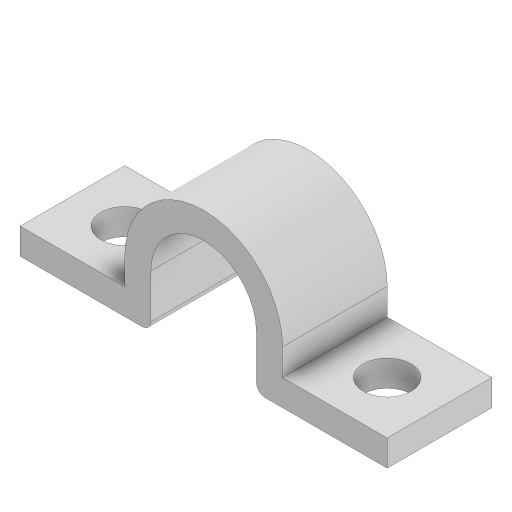
# Autodesk Inventor part: Pipe Clamp
Saved by Autodesk Inventor 2024 (Build 280153000, 153)
## iProperties
Created: 2025-04-26
Part Number: Pipe Clamp
Material: Generic
Document SubType Name: Modeling
Designer: Binara
Density: 1 g/cm^3
Appearance: Default
Author: Binara
Autodesk Inventor part; units mm, degrees
ref_plane "YZ Plane" through (0, 0, 0) normal (1, 0, 0) x (0, 1, 0)
ref_plane "XZ Plane" through (0, 0, 0) normal (0, 1, 0) x (-1, 0, 0)
ref_plane "XY Plane" through (0, 0, 0) normal (0, 0, 1) x (1, 0, 0)
sketch "Sketch1" plane through (0, 0, 0) normal (0, 0, 1) x (1, 0, 0)
  circle A0 centre (0, 0) radius 6.05
  circle A1 centre (0, 0) radius 9.05
  line L0 (-21.05, -6.05) -> (21.05, -6.05)
  line L1 (-9.05, 0) -> (-9.05, -6.05)
  line L2 (-6.05, 0) -> (-6.05, -6.05)
  line L3 (6.05, 0) -> (6.05, -6.05)
  line L4 (9.05, 0) -> (9.05, -6.05)
  line L5 (21.05, -6.05) -> (21.05, -3.05)
  line L6 (21.05, -3.05) -> (9.05, -3.05)
  line L7 (-21.05, -6.05) -> (-21.05, -3.05)
  line L8 (-21.05, -3.05) -> (-9.05, -3.05)
  dimension "d0" = 12.1
  dimension "d1" = 3
  dimension "d2" = 12
  dimension "d3" = 3
  dimension "d4" = 3
  dimension "d5" = 12
  constraints: 18 end point, 6 perpendicular, 6 point on line, 5 tangent, 4 point on circle, 2 centre point, 2 vertical, 1 coincident, 1 horizontal
  measures "d0" diameter of A0
  measures "d1" radial gap between concentric circles of A0 A1
  measures "d2" distance of L5.end L6.end
  measures "d3" distance of L0.end L5.end
  measures "d4" distance of L0.start L7.end
  measures "d5" distance of L7.end L8.end
extrude "Extrusion1" add sketch "Sketch1" along normal blind 12 contours A0 L2 L0 A1 L3 | A1 L4 L0 | L0 L1 A1 | L4 L6 L5 L0 | L0 L7 L8 L1
fillet "Fillet1" radius 1 2 edges at (6.05, -6.05, 6) (-6.05, -6.05, 6)
sketch "Sketch2" plane through (9.05, -3.05, 0) normal (0, 1, 0) x (1, 0, 0)
  line L0 (12, 0) -> (12, -12) projected
  line L1 (12, -6) -> (0, -6)
  line L2 (0, 0) -> (0, -12) projected
  line L3 (-18.1, -12) -> (0, -12) projected
  line L4 (-9.05, -12) -> (-9.05, -16.2316)
  circle A0 centre (6, -6) radius 2.75
  circle A1 centre (-24.1, -6) radius 2.75
  point P0 (-9.05, 0)
  dimension "d9" = 5.5
  constraints: 4 end point, 4 midpoint, 2 centre point, 1 symmetric about line, 1 vertical, 1 other
  measures "d9" diameter of A0
extrude "Extrusion2" cut sketch "Sketch2" against normal blind 12
equation "\"d4\" = d3"
equation "\"d5\" = d2"
body "Solid1"
